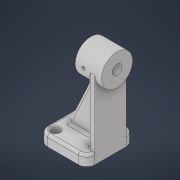
# Autodesk Inventor part: 1
Saved by Autodesk Inventor 2022 (Build 260153000, 153)
## iProperties
Created: 2022-09-05
Part Number: 1
Material: 일반
Document SubType Name: Modeling
Designer: USER
Density: 1 g/cm^3
Appearance: 기본값
Author: USER
Autodesk Inventor part; units mm, degrees
sketch "스케치1" plane through (0, 0, 0) normal (0, 0, 1) x (1, 0, 0)
  point P0 (0, 0)
sketch "스케치2" plane through (0, 0, 0) normal (0, 1, 0) x (-1, 0, 0)
  line L0 (28, 29) -> (-30, 29)
  line L1 (-30, 29) -> (-30, -29)
  line L2 (-30, -29) -> (28, -29)
  line L3 (28, -29) -> (28, 29)
  point P0 (0, 0)
  dimension "d0" = 29
  dimension "d1" = 58
  dimension "d2" = 58
  dimension "d3" = 28
  constraints: 8 end point, 2 parallel, 1 horizontal, 1 perpendicular
  measures "d0" distance from line of L0 point (0, 0)
  measures "d1" distance between parallel lines of L2 L0
  measures "d2" distance between parallel lines of L3 L1
  measures "d3" distance from line of point (0, 0) L3
extrude "돌출1" add sketch "스케치2" along normal blind 13
fillet "모깎기1" radius 10 4 edges at (30, 6.5, 29) (30, 6.5, -29) (-28, 6.5, -29) (-28, 6.5, 29)
sketch "스케치3" plane through (0, 13, 0) normal (0, 1, 0) x (1, 0, 0)
  line L0 (30, -19) -> (30, 19) projected
  line L1 (30, 19) -> (22, 19)
  line L2 (22, 19) -> (22, -19)
  line L3 (22, -19) -> (30, -19)
  line L4 (30, -19) -> (30, 19)
  point P0 (0, 0)
  dimension "d7" = 8
  constraints: 8 end point, 2 parallel, 1 horizontal, 1 perpendicular
  measures "d7" distance of L2.end L3.end
extrude "돌출2" add sketch "스케치3" along normal blind 82
fillet "모깎기2" radius 3 7 edges at (-25.0711, 13, 26.0711) (1, 13, 29) (27.0711, 13, 26.0711) (-25.0711, 13, -26.0711) (1, 13, -29) (27.0711, 13, -26.0711) (-28, 13, 0)
sketch "스케치4" plane through (0, 13, 0) normal (0, 1, 0) x (1, 0, 0)
  arc A0 (-18, 29) -> (-28, 19) centre (-18, 19) ccw projected
  circle A1 centre (-18, 19) radius 5
  arc A2 (-28, -19) -> (-18, -29) centre (-18, -19) ccw projected
  circle A3 centre (-18, -19) radius 5
  circle A4 centre (-18, -19) radius 5.5
  circle A5 centre (-18, 19) radius 5.5
  point P0 (0, 0)
  dimension "d11" = 10
  dimension "d12" = 10
  dimension "d13" = 11
  dimension "d14" = 11
  constraints: 4 centre point, 4 coincident
  measures "d11" diameter of A1
  measures "d12" diameter of A3
  measures "d13" diameter of A4
  measures "d14" diameter of A5
extrude "돌출3" cut sketch "스케치4" against normal through all contours A1 | A3
sketch "스케치5" plane through (22, 13, -19) normal (-1, 0, 0) x (0, 0, 1)
  point P0 (19, -13)
ref_plane "작업 평면1" through (26, 0, 19) normal (1, 0, 0) x (0, 0, -1)
sketch "스케치6" plane through (26, 0, 19) normal (1, 0, 0) x (0, 0, -1)
  line L0 (0, 95) -> (38, 95) projected
  circle A0 centre (19, 95) radius 19
  line L1 (42.1779, 114) -> (-32.8431, 114)
  point P0 (19, 0)
  dimension "d17" = 38
  constraints: 2 end point, 1 centre point, 1 horizontal, 1 midpoint
  measures "d17" diameter of A0
extrude "돌출4" add sketch "스케치6" along normal blind 12 and the other way blind 20
ref_plane "작업 평면2" through (-25, 13, 0) normal (0, 0, -1) x (-1, 0, 0)
sketch "스케치7" plane through (-25, 13, 0) normal (0, 0, -1) x (-1, 0, 0)
  line L0 (-31, 63) -> (-63, 63) projected
  line L1 (-36, 63) -> (-7, 0)
  line L2 (-7, 0) -> (-45, 0) projected
  line L3 (-52, 0) -> (-47, 0) projected
  line L4 (-7, 0) -> (-47, 0)
  line L5 (-47, 0) -> (-47, 63)
  line L6 (-47, 0) -> (-47, 82) projected
  point P0 (-25, -13)
  point P1 (3, -3)
  dimension "d22" = 5
  dimension "d23" = 10
  constraints: 6 end point, 3 point on line, 2 coincident, 1 horizontal, 1 midpoint
  measures "d22" distance of L1.start L0.start
  measures "d23" horizontal distance of point (3, -3) L1.end
extrude "돌출5" add sketch "스케치7" along normal mid plane 8
fillet "모깎기3" radius 3 10 edges at (-3.5, 44.5, 4) (22, 44.5, 4) (2, 13, 4) (22, 13, 11.5) (2, 13, -4) (22, 13, -11.5) (22, 44.5, -4) (-3.5, 44.5, -4) (22, 54, -19) (22, 54, 19)
sketch "스케치8" plane through (6, 95, 0) normal (-1, 0, 0) x (0, 0, 1)
  circle A0 centre (0, 0) radius 6.5
  circle A1 centre (0, 0) radius 6
  point P0 (0, -95)
  dimension "d27" = 13
  dimension "d28" = 12
  constraints: 2 centre point, 1 coincident
  measures "d27" diameter of A0
  measures "d28" diameter of A1
extrude "돌출6" cut sketch "스케치8" against normal blind 1 contours A0 | A1
extrude "돌출7" cut sketch "스케치8" against normal through all contours A1
ref_plane "작업 평면3" through (30, 10, 0) normal (0, 0, 1) x (1, 0, 0)
sketch "스케치9" plane through (30, 10, 0) normal (0, 0, 1) x (1, 0, 0)
  circle A0 centre (-14, 85) radius 2
  line L0 (8, 91) -> (8, 79) projected
  point P0 (-30, -10)
  dimension "d33" = 4
  dimension "d34" = 22
  constraints: 1 centre point
  measures "d33" diameter of A0
  measures "d34" distance from line of L0 A0.centre
extrude "돌출8" cut sketch "스케치9" along normal through all both and the other way through all
chamfer "모따기1" distance 1 angle 45 2 edges at (-23, 13, -19) (-23, 13, 19)
